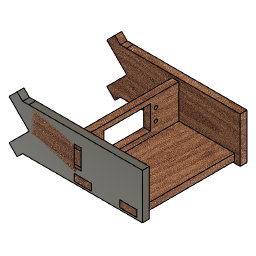
Gordijn v4 v3 (Autodesk Fusion 360 design; units mm, degrees)
Autodesk Fusion 360 part; units mm, degrees
sketch "Sketch1" plane through (0, 0, 0) normal (0, 1, 0) x (1, 0, 0)
  line L0 (159.0177, -128.1917) -> (159.0174, -88.1918)
  line L1 (159.0174, -88.1918) -> (59.0178, -88.1918)
  line L2 (59.0178, -88.1918) -> (59.0178, -88.1942)
  line L3 (59.0178, -88.1942) -> (53.5318, -88.1942)
  line L4 (53.5318, -88.1942) -> (53.5318, -88.3036)
  line L5 (53.5318, -88.3036) -> (48.6892, -83.4607)
  line L6 (48.6892, -83.4607) -> (41.6178, -90.5314)
  line L7 (41.6178, -90.5314) -> (59.0178, -107.9314)
  line L8 (59.0178, -107.9314) -> (59.0178, -108.4867)
  line L9 (59.0178, -108.4867) -> (41.6181, -125.8867)
  line L10 (41.6181, -125.8867) -> (48.6892, -132.9577)
  line L11 (48.6892, -132.9577) -> (53.4753, -128.1713)
  line L12 (53.4753, -128.1713) -> (59.0178, -128.1713)
  line L13 (59.0178, -128.1713) -> (59.0178, -128.191)
  line L14 (59.0178, -128.191) -> (159.0177, -128.1917)
  line L15 (139.0177, -120.5837) -> (154.0178, -120.5837)
  line L16 (154.0178, -120.5837) -> (154.0178, -126.5841)
  line L17 (154.0178, -126.5841) -> (139.0177, -126.5841)
  line L18 (139.0177, -126.5841) -> (139.0177, -120.5837)
  line L19 (99.0181, -120.5837) -> (114.0182, -120.5837)
  line L20 (114.0182, -120.5837) -> (114.0182, -126.5841)
  line L21 (114.0182, -126.5841) -> (99.0181, -126.5841)
  line L22 (99.0181, -126.5841) -> (99.0181, -120.5837)
  line L23 (99.0181, -100.6917) -> (105.0185, -100.6917)
  line L24 (105.0185, -100.6917) -> (105.0185, -115.6918)
  line L25 (105.0185, -115.6918) -> (99.0181, -115.6918)
  line L26 (99.0181, -115.6918) -> (99.0181, -100.6917)
extrude "Extrude1" add sketch "Sketch1" along normal blind 6 makes body 1
copy_body "CopyPasteBodies1" bodies 1 makes body 2
move_body "Move1" bodies 2 to x (1, 0, 0) y (0, 1, 0) z (0, 0, 1) at (0, 90, 0)
move_body "Move2" bodies 1 to x (1, 0, 0) y (0, -1, 0) z (0, 0, -1) at (0, 0, 166.9213)
move_body "Move3" bodies 2 to x (1, 0, 0) y (0, -1, 0) z (0, 0, -1) at (0, 180, 166.9213)
sketch "Sketch2" plane through (0, 0, 0) normal (0, 0, 1) x (1, 0, 0)
  line L0 (133.6132, -84.6703) -> (133.6132, -69.6703)
  line L1 (133.6132, -69.6703) -> (127.6128, -69.6703)
  line L2 (127.6128, -69.6703) -> (122.6136, -69.6703)
  line L3 (122.6136, -69.6703) -> (122.6136, -75.6703)
  line L4 (122.6136, -75.6703) -> (107.6139, -75.6703)
  line L5 (107.6139, -75.6703) -> (107.6139, -69.6703)
  line L6 (107.6139, -69.6703) -> (67.6129, -69.6703)
  line L7 (67.6129, -69.6703) -> (67.6129, -75.6703)
  line L8 (67.6129, -75.6703) -> (52.6128, -75.6703)
  line L9 (52.6128, -75.6703) -> (52.6128, -69.6703)
  line L10 (52.6128, -69.6703) -> (47.6132, -69.6703)
  line L11 (47.6132, -69.6703) -> (41.6132, -69.6703)
  line L12 (41.6132, -69.6703) -> (41.6132, -84.6703)
  line L13 (41.6132, -84.6703) -> (47.6132, -84.6703)
  line L14 (47.6132, -84.6703) -> (47.6132, -109.6702)
  line L15 (47.6132, -109.6702) -> (41.6132, -109.6702)
  line L16 (41.6132, -109.6702) -> (41.6132, -124.6699)
  line L17 (41.6132, -124.6699) -> (47.6132, -124.6699)
  line L18 (47.6132, -124.6699) -> (53.6133, -124.6699)
  line L19 (53.6133, -124.6699) -> (121.6128, -124.6699)
  line L20 (121.6128, -124.6699) -> (127.6128, -124.6699)
  line L21 (127.6128, -124.6699) -> (133.6132, -124.6699)
  line L22 (133.6132, -124.6699) -> (133.6132, -109.6702)
  line L23 (133.6132, -109.6702) -> (127.6128, -109.6702)
  line L24 (127.6128, -109.6702) -> (127.6128, -84.6703)
  line L25 (127.6128, -84.6703) -> (133.6132, -84.6703)
extrude "Extrude2" add sketch "Sketch2" along normal blind 6 separate body makes body 3
copy_body "Body->Comp1" bodies 1 removing the originals makes body 4 in component "Component"
copy_body "Body->Comp2" bodies 2 removing the originals makes body 5 in component "Component'"
copy_body "Body->Comp3" bodies 3 removing the originals makes body 6 in component "Component''"
sketch "Sketch3" plane through (0, 0, 0) normal (0, 0, 1) x (1, 0, 0)
  line L0 (153.1002, -85.7883) -> (147.1006, -85.7883)
  line L1 (147.1006, -85.7883) -> (147.1006, -78.2882)
  line L2 (147.1006, -78.2882) -> (67.101, -78.2882)
  line L3 (67.101, -78.2882) -> (67.101, -85.7883)
  line L4 (67.101, -85.7883) -> (61.101, -85.7883)
  line L5 (61.101, -85.7883) -> (61.101, -100.788)
  line L6 (61.101, -100.788) -> (67.101, -100.788)
  line L7 (67.101, -100.788) -> (67.101, -108.288)
  line L8 (67.101, -108.288) -> (71.1001, -108.288)
  line L9 (71.1001, -108.288) -> (71.1001, -114.2881)
  line L10 (71.1001, -114.2881) -> (86.0998, -114.2881)
  line L11 (86.0998, -114.2881) -> (86.0998, -108.288)
  line L12 (86.0998, -108.288) -> (126.1008, -108.288)
  line L13 (126.1008, -108.288) -> (126.1008, -114.2881)
  line L14 (126.1008, -114.2881) -> (141.1009, -114.2881)
  line L15 (141.1009, -114.2881) -> (141.1009, -108.288)
  line L16 (141.1009, -108.288) -> (147.1006, -108.288)
  line L17 (147.1006, -108.288) -> (147.1006, -100.788)
  line L18 (147.1006, -100.788) -> (153.1002, -100.788)
  line L19 (153.1002, -100.788) -> (153.1002, -85.7883)
  line L20 (81.1468, -82.7886) -> (122.1469, -82.7886)
  line L21 (122.1469, -82.7886) -> (122.1469, -103.7884)
  line L22 (122.1469, -103.7884) -> (81.1468, -103.7884)
  line L23 (81.1468, -103.7884) -> (81.1468, -82.7886)
  circle A0 centre (126.8829, -88.0782) radius 1.5
  circle A1 centre (126.8829, -98.3983) radius 1.5
  circle A2 centre (76.3473, -88.129) radius 1.5
  circle A3 centre (76.3473, -98.4491) radius 1.5
  point P0 (128.3829, -88.0782)
  point P1 (128.3829, -98.3983)
  point P2 (77.8473, -88.129)
  point P3 (77.8473, -98.4491)
extrude "Extrude3" add sketch "Sketch3" along normal blind 6 separate body makes body 7
copy_body "Body->Comp4" bodies 7 removing the originals makes body 8 in component "Component'''"
sketch "Sketch4" plane through (0, 0, 0) normal (0, 1, 0) x (1, 0, 0)
  line L0 (159.0177, -128.1917) -> (159.0174, -88.1918)
  line L1 (159.0174, -88.1918) -> (59.0178, -88.1918)
  line L2 (59.0178, -88.1918) -> (59.0178, -88.1942)
  line L3 (59.0178, -88.1942) -> (53.5318, -88.1942)
  line L4 (53.5318, -88.1942) -> (53.5318, -88.3036)
  line L5 (53.5318, -88.3036) -> (48.6892, -83.4607)
  line L6 (48.6892, -83.4607) -> (41.6178, -90.5314)
  line L7 (41.6178, -90.5314) -> (59.0178, -107.9314)
  line L8 (59.0178, -107.9314) -> (59.0178, -108.4867)
  line L9 (59.0178, -108.4867) -> (41.6181, -125.8867)
  line L10 (41.6181, -125.8867) -> (48.6892, -132.9577)
  line L11 (48.6892, -132.9577) -> (53.4753, -128.1713)
  line L12 (53.4753, -128.1713) -> (59.0178, -128.1713)
  line L13 (59.0178, -128.1713) -> (59.0178, -128.191)
  line L14 (59.0178, -128.191) -> (159.0177, -128.1917)
  line L15 (139.0177, -120.5837) -> (154.0178, -120.5837)
  line L16 (154.0178, -120.5837) -> (154.0178, -126.5841)
  line L17 (154.0178, -126.5841) -> (139.0177, -126.5841)
  line L18 (139.0177, -126.5841) -> (139.0177, -120.5837)
  line L19 (99.0181, -120.5837) -> (114.0182, -120.5837)
  line L20 (114.0182, -120.5837) -> (114.0182, -126.5841)
  line L21 (114.0182, -126.5841) -> (99.0181, -126.5841)
  line L22 (99.0181, -126.5841) -> (99.0181, -120.5837)
  line L23 (99.0181, -98.0843) -> (105.0185, -98.0843)
  line L24 (105.0185, -98.0843) -> (105.0185, -113.0844)
  line L25 (105.0185, -113.0844) -> (99.0181, -113.0844)
  line L26 (99.0181, -113.0844) -> (99.0181, -98.0843)
extrude "Extrude4" add sketch "Sketch4" along normal blind 6 separate body makes body 9
move_body "Move4" bodies 9 to x (1, 0, 0) y (0, -1, 0) z (0, 0, -1) at (0, 12, 226.1688)
copy_body "CopyPasteBodies2" bodies 9 makes body 10
move_body "Move5" bodies 10 to x (1, 0, 0) y (0, 1, 0) z (0, 0, 1) at (0, 85, 0)
copy_body "Body->Comp5" bodies 9 removing the originals makes body 11 in component "Component''''"
copy_body "Body->Comp6" bodies 10 removing the originals makes body 12 in component "Component'''''"
sketch "Sketch5" plane through (0, 0, 0) normal (1, 0, 0) x (0, 1, 0)
  line L0 (153.1002, -85.7883) -> (147.1006, -85.7883)
  line L1 (147.1006, -85.7883) -> (147.1006, -78.4682)
  line L2 (147.1006, -78.4682) -> (67.101, -78.4682)
  line L3 (67.101, -78.4682) -> (67.101, -85.9682)
  line L4 (67.101, -85.9682) -> (60.9979, -85.9682)
  line L5 (60.9979, -85.9682) -> (60.9979, -100.9679)
  line L6 (60.9979, -100.9679) -> (67.101, -100.9679)
  line L7 (67.101, -100.9679) -> (67.101, -108.468)
  line L8 (67.101, -108.468) -> (72.0702, -108.468)
  line L9 (72.0702, -108.468) -> (72.0702, -114.468)
  line L10 (72.0702, -114.468) -> (87.0699, -114.468)
  line L11 (87.0699, -114.468) -> (87.0699, -108.468)
  line L12 (87.0699, -108.468) -> (127.1034, -108.468)
  line L13 (127.1034, -108.468) -> (127.1034, -114.6377)
  line L14 (127.1034, -114.6377) -> (142.1031, -114.6377)
  line L15 (142.1031, -114.6377) -> (142.1031, -108.468)
  line L16 (142.1031, -108.468) -> (147.1006, -108.468)
  line L17 (147.1006, -108.468) -> (147.1006, -100.788)
  line L18 (147.1006, -100.788) -> (153.1002, -100.788)
  line L19 (153.1002, -100.788) -> (153.1002, -85.7883)
  line L20 (81.1468, -82.7886) -> (122.1469, -82.7886)
  line L21 (122.1469, -82.7886) -> (122.1469, -103.7884)
  line L22 (122.1469, -103.7884) -> (81.1468, -103.7884)
  line L23 (81.1468, -103.7884) -> (81.1468, -82.7886)
  circle A0 centre (126.8829, -88.0782) radius 1.5
  circle A1 centre (126.8829, -98.3983) radius 1.5
  circle A2 centre (76.3473, -88.129) radius 1.5
  circle A3 centre (76.3473, -98.4491) radius 1.5
  point P0 (128.3829, -88.0782)
  point P1 (128.3829, -98.3983)
  point P2 (77.8473, -88.129)
  point P3 (77.8473, -98.4491)
extrude "Extrude5" add sketch "Sketch5" along normal blind 6 separate body makes body 13
copy_body "Body->Comp7" bodies 13 removing the originals makes body 14 in component "Component''''''"
component "Component" placed x (1, 0, 0) y (0, 1, 0) z (0, 0, 1) at (0, 0, 0)
component "Component'" placed x (1, 0, 0) y (0, 1, 0) z (0, 0, 1) at (-0.0002, -4, -0.0002)
component "Component''" placed x (0, 1, 0) y (-1, 0, 0) z (0, 0, 1) at (29.3477, -47.6132, 40.3372)
component "Component'''" placed x (0, -1, 0) y (0, 0, 1) z (-1, 0, 0) at (105.0183, 147.1009, 154.6249)
component "Component''''" placed x (1, 0, 0) y (0, 1, 0) z (0, 0, 1) at (0, -12, -59.2475)
component "Component'''''" placed x (1, 0, 0) y (0, 1, 0) z (0, 0, 1) at (0, -11, -59.2475)
component "Component''''''" placed x (1, 0, 0) y (0, 1, 0) z (0, 0, 1) at (99.018, -67.0704, 154.8052)
